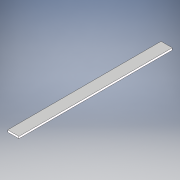
# Autodesk Inventor part: 56 in k wool
Saved by Autodesk Inventor 2017 (Build 210142000, 142)
## iProperties
Created: 2017-06-22
Part Number: 56 in k wool
Material: Generic
Document SubType Name: Modeling
Designer: cas7
Density: 1 g/cm^3
Appearance: Default
Author: cas7
Autodesk Inventor part; units mm, degrees
ref_plane "YZ Plane" through (0, 0, 0) normal (1, 0, 0) x (0, 1, 0)
ref_plane "XZ Plane" through (0, 0, 0) normal (0, 1, 0) x (-1, 0, 0)
ref_plane "XY Plane" through (0, 0, 0) normal (0, 0, 1) x (1, 0, 0)
sketch "Sketch1" plane through (0, 0, 0) normal (0, 1, 0) x (-1, 0, 0)
  line L0 (0, 0) -> (88.9, 0)
  line L1 (88.9, 0) -> (88.9, -1422.4)
  line L2 (88.9, -1422.4) -> (0, -1422.4)
  line L3 (0, -1422.4) -> (0, 0)
  dimension "d0" = 88.9
  dimension "d1" = 1422.4
  constraints: 8 end point, 2 parallel, 1 horizontal, 1 perpendicular
  measures "d0" distance of L1.end L2.end
  measures "d1" distance of L0.end L1.end
extrude "Extrusion1" add sketch "Sketch1" along normal blind 3.175
sketch "Sketch2" plane through (0, 0, 0) normal (1, 0, 0) x (0, 0, -1)
  line L0 (1422.4, 0) -> (0, 0) projected
  line L1 (1422.4, 0) -> (1422.4, 3.175) projected
  line L2 (0, 3.175) -> (1422.4, 3.175) projected
  line L3 (0, 0) -> (0, 3.175) projected
extrude "Extrusion2" add sketch "Sketch2" along normal blind 15.875
sketch "Sketch3" plane through (-88.9, 0, -1422.4) normal (0, 0, -1) x (-1, 0, 0)
  line L0 (0, 0) -> (-104.775, 0) projected
  line L1 (0, 0) -> (0, 3.175) projected
  line L2 (0, 3.175) -> (-104.775, 3.175) projected
  line L3 (-104.775, 0) -> (-104.775, 3.175) projected
  point P0 (-88.9, 0)
extrude "Extrusion3" add sketch "Sketch3" along normal blind 6.35
sketch "Sketch4" plane through (0, 3.175, 0) normal (0, 1, 0) x (1, 0, 0)
  line L0 (-88.9, 0) -> (15.875, 0) projected
  line L1 (15.875, 0) -> (15.875, 1428.75) projected
  line L2 (-88.9, 1428.75) -> (15.875, 1428.75) projected
  line L3 (-88.9, 0) -> (-88.9, 1428.75) projected
  point P0 (0, 0)
extrude "Extrusion4" add sketch "Sketch4" along normal blind 15.875
body "Solid1"
